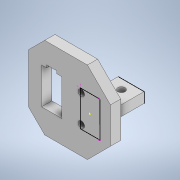
# Autodesk Inventor part: Servo Holder Module
Saved by Autodesk Inventor 2020 (Build 240168000, 168)
## iProperties
Created: 2020-03-03
Part Number: Servo Holder Module
Material: Generic
Document SubType Name: Modeling
Designer: Varun Kumar
Density: 1 g/cm^3
Appearance: Default
Author: Varun Kumar
Autodesk Inventor part; units mm, degrees
ref_plane "YZ Plane" through (0, 0, 0) normal (1, 0, 0) x (0, 1, 0)
ref_plane "XZ Plane" through (0, 0, 0) normal (0, 1, 0) x (-1, 0, 0)
ref_plane "XY Plane" through (0, 0, 0) normal (0, 0, 1) x (1, 0, 0)
sketch "Sketch1" plane through (0, 0, 0) normal (0, 0, 1) x (1, 0, 0)
  line L0 (-38.1, -25.4) -> (38.1, -25.4)
  line L1 (38.1, -25.4) -> (38.1, 25.4)
  line L2 (38.1, 25.4) -> (-38.1, 25.4)
  line L3 (-38.1, 25.4) -> (-38.1, -25.4)
  line L4 (-38.1, -25.4) -> (38.1, 25.4) construction
  line L5 (38.1, -25.4) -> (-38.1, 25.4) construction
  point P0 (0, 0)
  dimension "d0" = 76.2
  dimension "d1" = 50.8
  constraints: 12 end point, 2 midpoint, 2 parallel, 1 horizontal, 1 perpendicular
  measures "d0" distance of L2.end L1.end
  measures "d1" distance of L1.end L0.end
extrude "Extrusion1" add sketch "Sketch1" along normal blind 6.35
sketch "Sketch3" plane through (38.1, -25.4, 0) normal (1, 0, 0) x (0, 0, -1)
  line L0 (0, 0) -> (0, 50.8) projected
  line L1 (0, 50.8) -> (-6.35, 50.8) projected
  line L2 (-6.35, 0) -> (-6.35, 50.8) projected
  line L3 (0, 0) -> (-6.35, 0) projected
  point P0 (0, 25.4)
extrude "Extrusion3" cut sketch "Sketch3" against normal blind 25.4
sketch "Sketch4" plane through (-38.1, -25.4, 0) normal (-1, 0, 0) x (0, 0, 1)
  line L0 (4.925, 17.15) -> (1.425, 17.15)
  line L1 (1.425, 17.15) -> (1.425, 33.65)
  line L2 (1.425, 33.65) -> (4.925, 33.65)
  line L3 (4.925, 33.65) -> (4.925, 17.15)
  line L4 (4.925, 17.15) -> (1.425, 33.65) construction
  line L5 (1.425, 17.15) -> (4.925, 33.65) construction
  point P0 (0, 25.4)
  point P1 (3.175, 25.4)
  dimension "d9" = 3.5
  dimension "d10" = 16.5
  constraints: 12 end point, 2 midpoint, 2 parallel, 1 horizontal, 1 perpendicular
  measures "d9" distance of L1.end L2.end
  measures "d10" distance of L0.end L1.end
extrude "Extrusion4" add sketch "Sketch4" along normal blind 3.302
sketch "Sketch5" plane through (-38.1, -8.25, 4.925) normal (0, 0, 1) x (1, 0, 0)
  line L0 (-3.302, 0) -> (-3.302, 16.5) projected
  line L1 (0, 16.5) -> (0, 0) projected
  line L2 (0, 16.5) -> (-3.302, 16.5) projected
  line L3 (-3.302, 0) -> (-3.302, 16.5) projected
  line L4 (0, 0) -> (-3.302, 0) projected
  line L5 (-3.302, 16.5) -> (-3.175, 16.5)
  line L6 (0, 16.5) -> (-3.302, 16.5) projected
  line L7 (-3.175, 16.5) -> (-3.175, 16.5685)
  line L8 (-3.302, 16.5) -> (-3.302, 0) projected
  line L9 (-3.175, 16.5685) -> (-3.302, 16.5)
  point P0 (38.1, 8.25)
  point P1 (-3.175, 16.5)
  dimension "d13" = 0.127
  constraints: 6 end point, 1 perpendicular, 1 point on line
  measures "d13" distance of L2.end L5.end
sketch3d "3D Sketch1"
  line L0 (-41.402, 8.25, 4.925) -> (-41.402, 8.25, 1.425)
  line L1 (-41.402, 8.25, 1.425) -> (-41.402, -8.25, 1.425)
  line L2 (-41.402, -8.25, 1.425) -> (-41.402, -8.25, 4.925)
  line L3 (-41.402, -8.25, 4.925) -> (-41.402, 8.25, 4.925)
sweep "Sweep1" add profiles "Sketch5" path "3D Sketch1" contours L9 L7 L2
chamfer "Chamfer1" distance 14.2875 angle 45 4 edges at (-38.1, -25.4, 3.175) (-38.1, 25.4, 3.175) (12.7, -25.4, 3.175) (12.7, 25.4, 3.175)
sketch "Sketch6" plane through (-41.402, -25.4, 0) normal (-1, 0, 0) x (0, 0, 1)
  line L0 (-26.5368, -66.9991) -> (26.5368, -66.9991)
  line L1 (26.5368, -66.9991) -> (26.5368, 66.9991)
  line L2 (26.5368, 66.9991) -> (-26.5368, 66.9991)
  line L3 (-26.5368, 66.9991) -> (-26.5368, -66.9991)
  line L4 (0, 0) -> (6.35, 0) projected
  line L5 (-26.5368, -66.9991) -> (26.5368, 66.9991) construction
  line L6 (26.5368, -66.9991) -> (-26.5368, 66.9991) construction
  point P0 (0, 25.4)
  constraints: 12 end point, 2 midpoint, 2 parallel, 1 horizontal, 1 perpendicular
extrude "Extrusion5" cut sketch "Sketch6" against normal blind 28.575
sketch "Sketch7" plane through (0, 0, 0) normal (0, 0, -1) x (-1, 0, 0)
  line L0 (-8.025, 3.175) -> (-8.025, -3.175)
  line L1 (-8.025, -3.175) -> (8.025, -3.175)
  line L2 (8.025, -3.175) -> (8.025, 3.175)
  line L3 (8.025, 3.175) -> (-8.025, 3.175)
  line L4 (-8.025, 4.675) -> (8.025, -1.675) construction
  line L5 (-8.025, -1.675) -> (8.025, 4.675) construction
  line L6 (0, 3.175) -> (0, -3.175)
  point P0 (0, 0)
  point P1 (0, 0)
  dimension "d21" = 6.35
  dimension "d22" = 16.05
  constraints: 14 end point, 2 parallel, 1 midpoint, 1 perpendicular
  measures "d21" distance of L2.end L1.end
  measures "d22" distance of L1.end L0.end
extrude "Extrusion6" add sketch "Sketch7" along normal blind 19.2024
sketch "Sketch9" plane through (0, 0, 6.35) normal (0, 0, 1) x (1, 0, 0)
  line L0 (6.0307, -10.9832) -> (5.9693, 11.0167) projected
  line L1 (-6.0307, 10.9832) -> (6.0307, 10.9832)
  line L2 (6.0307, 10.9832) -> (6.0307, -10.9832)
  line L3 (6.0307, -10.9832) -> (-6.0307, -10.9832)
  line L4 (-6.0307, -10.9832) -> (-6.0307, 10.9832)
  point P0 (0, 0)
  constraints: 8 end point, 2 parallel, 1 horizontal, 1 perpendicular
sketch "Sketch10" plane through (-12.827, -25.4, 0) normal (-1, 0, 0) x (0, 0, 1)
  line L0 (0, 0) -> (0, 50.8) projected
  line L1 (6.35, 0) -> (0, 0) projected
  line L2 (6.35, 50.8) -> (6.35, 0) projected
  line L3 (0, 50.8) -> (6.35, 50.8) projected
  point P0 (0, 25.4)
extrude "Extrusion7" add sketch "Sketch10" along normal blind 25.4
chamfer "Chamfer2" distance 10.16 angle 45 1 edges at (-38.227, 25.4, 3.175)
chamfer "Chamfer3" distance 10.16 angle 45 1 edges at (-38.227, -25.4, 3.175)
sketch "Sketch11" plane through (0, 0, 6.35) normal (0, 0, 1) x (1, 0, 0)
  line L0 (-29.728, 10.9832) -> (-17.6666, 10.9832)
  line L1 (-17.6666, -10.9832) -> (-29.728, -10.9832)
  line L2 (-29.728, -10.9832) -> (-29.728, 10.9832)
  line L3 (-17.6666, -10.9832) -> (-17.6666, 10.9832)
  line L4 (-30.998, 12.2532) -> (-16.3966, 12.2532)
  line L5 (-16.3966, 12.2532) -> (-16.3966, -12.2532)
  line L6 (-16.3966, -12.2532) -> (-30.998, -12.2532)
  line L7 (-30.998, -12.2532) -> (-30.998, 12.2532)
  line L8 (-17.6666, 10.9832) -> (-18.9366, 10.9832)
  line L9 (-29.728, 10.9832) -> (-28.458, 10.9832)
  line L10 (-18.9366, 10.9832) -> (-28.458, 10.9832)
  line L11 (-28.458, 10.9832) -> (-28.458, 15.1856)
  line L12 (-28.458, 15.1856) -> (-18.9366, 15.1856)
  line L13 (-18.9366, 15.1856) -> (-18.9366, 10.9832)
  point P0 (0, 0)
  dimension "d54" = 1.27
  dimension "d55" = 1.27
  dimension "d56" = 1.27
  constraints: 28 end point, 4 parallel, 3 perpendicular, 2 horizontal, 2 point on line, 1 coincident, 3 other
  measures "d54" distance between parallel lines of L2 L7
  measures "d55" distance of L0.end L8.end
  measures "d56" distance of L2.end L9.end
extrude "Extrusion8" cut sketch "Sketch11" against normal up to surface (6.35 mm away) contours L0 L3 L1 L2
sketch "Sketch12" plane through (0, 0, 6.35) normal (0, 0, 1) x (1, 0, 0)
  arc A0 (-5.2182, -6.4143) -> (-5.5402, -10.4006) centre (-5.418, -8.4043) ccw projected
  arc A1 (-5.5402, -10.4006) -> (-5.2182, -6.4143) centre (-5.3404, -8.4106) ccw projected
  arc A2 (-5.3792, 10.6071) -> (-5.3792, 6.6078) centre (-5.418, 8.6074) ccw projected
  arc A3 (-5.3792, 6.6078) -> (-5.3792, 10.6071) centre (-5.3404, 8.6074) ccw projected
  line L0 (-14.078, 16.1258) -> (3.242, 16.1258) projected
  line L1 (-14.078, 16.1258) -> (-14.078, -15.929) projected
  line L2 (-14.078, -15.929) -> (3.242, -15.929) projected
  line L3 (3.242, 16.1258) -> (3.242, -15.929) projected
  circle A4 centre (-5.3404, -8.4106) radius 2
  circle A5 centre (-5.3404, 8.6074) radius 2
  point P0 (0, 0)
  point P1 (-5.3792, 6.6078)
  point P2 (-5.2182, -6.4143)
  point P3 (-5.5402, -10.4006)
  dimension "d38" = 4
  dimension "d39" = 4
  constraints: 2 centre point, 2 coincident
  measures "d38" diameter of A4
  measures "d39" diameter of A5
extrude "Extrusion9" cut sketch "Sketch12" against normal up to surface (6.35 mm away) contours A1 A4 | A3 A5
sketch "Sketch13" plane through (-8.025, 3.175, 0) normal (0, 1, 0) x (1, 0, 0)
  line L0 (16.05, 19.2024) -> (0, 19.2024) projected
  circle A0 centre (8.025, 4.3815) radius 2.25
  circle A1 centre (8.025, 13.1445) radius 2.25
  line L1 (16.05, 0) -> (0, 0) projected
  line L2 (16.05, 0) -> (16.05, 19.2024) projected
  line L3 (0, 19.2024) -> (16.05, 19.2024) projected
  line L4 (0, 0) -> (0, 19.2024) projected
  line L5 (8.025, 0) -> (12.4065, 0)
  line L6 (6.4375, 0) -> (20.725, 0) projected
  line L7 (8.025, 0) -> (8.025, 4.3815)
  line L8 (8.025, 0) -> (12.4065, 0) construction
  line L9 (8.025, 0) -> (21.1695, 0)
  line L10 (8.025, 0) -> (8.025, 13.1445)
  line L11 (16.05, 0) -> (0, 0) projected
  line L12 (8.025, 0) -> (21.1695, 0) construction
  dimension "d44" = 4.5
  dimension "d45" = 4.5
  dimension "d48" = 4.3815
  dimension "d49" = 4.3815
  dimension "d50" = 90
  dimension "d51" = 13.1445
  dimension "d52" = 13.1445
  dimension "d53" = 90
  constraints: 12 end point, 3 perpendicular, 2 centre point, 2 coincident, 2 horizontal, 2 point on line
  measures "d44" diameter of A0
  measures "d45" diameter of A1
  measures "d48" distance of L5.start L5.end
  measures "d49" distance of L5.start L7.end
  measures "d50" angle of L8 L7
  measures "d51" distance of L5.start L9.end
  measures "d52" distance of L5.start L10.end
  measures "d53" angle of L12 L10
extrude "Extrusion10" cut sketch "Sketch13" against normal up to surface (6.35 mm away) contours A1 | A0 L10 L7 | L7 L10 A0
sketch "Sketch14" plane through (0, 0, -19.2024) normal (0, 0, -1) x (-1, 0, 0)
  line L0 (8.025, 3.175) -> (8.025, -3.175) projected
  line L1 (-8.025, -3.175) -> (-8.025, 3.175) projected
  line L2 (8.025, 3.175) -> (-8.025, 3.175)
  line L3 (-8.025, 3.175) -> (-8.025, -3.175)
  line L4 (-8.025, -3.175) -> (8.025, -3.175)
  line L5 (8.025, -3.175) -> (8.025, 3.175)
  point P0 (0, 0)
  constraints: 8 end point, 2 parallel, 1 horizontal, 1 perpendicular
sketch "Sketch16" plane through (0, 0, 6.35) normal (0, 0, 1) x (1, 0, 0)
  line L0 (-29.728, -10.9832) -> (-29.728, 10.9832) projected
  line L1 (-17.6666, -10.9832) -> (-29.728, -10.9832) projected
  line L2 (-17.6666, 10.9832) -> (-17.6666, -10.9832) projected
  line L3 (-29.728, 10.9832) -> (-17.6666, 10.9832) projected
  line L4 (-29.982, -11.2372) -> (-29.982, 11.2372)
  line L5 (-29.982, 11.2372) -> (-17.4126, 11.2372)
  line L6 (-17.4126, 11.2372) -> (-17.4126, -11.2372)
  line L7 (-17.4126, -11.2372) -> (-29.982, -11.2372)
  point P0 (0, 0)
  dimension "d62" = 0.254
  constraints: 8 end point, 3 other
  measures "d62" distance between parallel lines of L1 L7
extrude "Extrusion12" cut sketch "Sketch16" against normal up to surface (6.35 mm away)
sketch "Sketch17" plane through (0, 0, 6.35) normal (0, 0, 1) x (1, 0, 0)
  line L0 (-17.4126, 11.2372) -> (-29.982, 11.2372) projected
  line L1 (-29.982, 11.2372) -> (-26.807, 11.2372)
  line L2 (-17.4126, 11.2372) -> (-20.5876, 11.2372)
  line L3 (-26.807, 11.2372) -> (-20.5876, 11.2372)
  line L4 (-20.5876, 11.2372) -> (-20.5876, 12.8247)
  line L5 (-20.5876, 12.8247) -> (-26.807, 12.8247)
  line L6 (-26.807, 12.8247) -> (-26.807, 11.2372)
  point P0 (0, 0)
  dimension "d65" = 3.175
  dimension "d66" = 3.175
  dimension "d67" = 1.5875
  constraints: 12 end point, 2 parallel, 2 point on line, 1 horizontal, 1 perpendicular
  measures "d65" distance of L0.end L1.end
  measures "d66" distance of L0.start L2.end
  measures "d67" distance of L4.end L3.end
extrude "Extrusion13" cut sketch "Sketch17" against normal up to surface (6.35 mm away)
body "Solid1"
